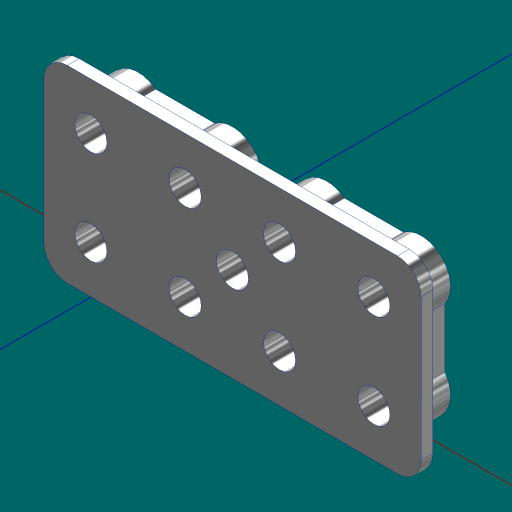
# Autodesk Inventor part: IntakeShoulder
Saved by Autodesk Inventor 2023.1 (Build 271208000, 208)
## iProperties
Created: 2022-11-06
Part Number: IntakeShoulder
Material: Aluminum 6061
Document SubType Name: Modeling
Designer: zac-h
Density: 2.7 g/cm^3
Appearance: Aluminum - Flat
Mass: 11.2632 g
Surface Area: 43.63 cm^2
Volume: 4.17154 cm^3
Author: zac-h
Autodesk Inventor part; units mm, degrees
ref_plane "YZ Plane" through (0, 0, 0) normal (1, 0, 0) x (0, 1, 0)
ref_plane "XZ Plane" through (0, 0, 0) normal (0, 1, 0) x (-1, 0, 0)
ref_plane "XY Plane" through (0, 0, 0) normal (0, 0, 1) x (1, 0, 0)
sketch "Sketch1" plane through (0, 0, 0) normal (0, 0, 1) x (1, 0, 0)
  circle A0 centre (0, 0) radius 2.159
  line L0 (0, 0) -> (38.1, 0) construction
  line L1 (0, 0) -> (0, 12.7) construction
  circle A1 centre (12.7, 0) radius 2.159
  circle A2 centre (25.4, 0) radius 2.159
  circle A3 centre (38.1, 0) radius 2.159
  circle A4 centre (0, 12.7) radius 2.159
  circle A5 centre (12.7, 12.7) radius 2.159
  circle A6 centre (25.4, 12.7) radius 2.159
  circle A7 centre (38.1, 12.7) radius 2.159
  circle A8 centre (19.05, 6.35) radius 2.159
  line L2 (12.7, 12.7) -> (25.4, 0) construction
  line L3 (-6.35, 19.05) -> (44.45, 19.05)
  line L4 (44.45, 19.05) -> (44.45, -6.35)
  line L5 (44.45, -6.35) -> (-6.35, -6.35)
  line L6 (-6.35, -6.35) -> (-6.35, 19.05)
  circle A9 centre (0, 12.7) radius 6.35 construction
  circle A10 centre (38.1, 0) radius 6.35 construction
  dimension "d0" = 4.318
  dimension "d1" = 38.1
  dimension "d9" = 12.7
  dimension "d12" = 12.7
  dimension "d15" = 12.7
  dimension "d18" = 4.318
  dimension "d19" = 25.4
  constraints: 14 end point, 11 centre point, 4 tangent, 3 coincident, 3 horizontal, 2 parallel, 2 vertical, 1 equal radius, 1 midpoint, 1 perpendicular, 14 other
  measures "d0" diameter of A0
  measures "d1" distance of L0.start L0.end
  measures "d9" distance of L0.start L1.end
  measures "d12" distance of L0.start A1.centre
  measures "d15" distance of L0.start A4.centre
  measures "d18" diameter of A8
  measures "d19" distance of L3.end L4.end
extrude "Extrusion1" add sketch "Sketch1" along normal blind 6.35
fillet "Fillet1" radius 3.175 4 edges at (44.45, 19.05, 3.175) (44.45, -6.35, 3.175) (-6.35, -6.35, 3.175) (-6.35, 19.05, 3.175)
sketch "Sketch2" plane through (0, 0, 0) normal (0, 0, -1) x (-1, 0, 0)
  arc A0 (6.35, 15.875) -> (3.175, 19.05) centre (3.175, 15.875) ccw projected
  line L0 (-41.275, 19.05) -> (3.175, 19.05) projected
  arc A1 (-41.275, 19.05) -> (-44.45, 15.875) centre (-41.275, 15.875) ccw projected
  line L1 (-44.45, -3.175) -> (-44.45, 15.875) projected
  arc A2 (-44.45, -3.175) -> (-41.275, -6.35) centre (-41.275, -3.175) ccw projected
  line L2 (3.175, -6.35) -> (-41.275, -6.35) projected
  arc A3 (3.175, -6.35) -> (6.35, -3.175) centre (3.175, -3.175) ccw projected
  line L3 (6.35, 15.875) -> (6.35, -3.175) projected
  circle A4 centre (-19.05, 6.35) radius 2.159 projected
  circle A5 centre (0, 0) radius 2.159 projected
  circle A6 centre (-12.7, 0) radius 2.159 projected
  circle A7 centre (-25.4, 0) radius 2.159 projected
  circle A8 centre (-38.1, 0) radius 2.159 projected
  circle A9 centre (0, 12.7) radius 2.159 projected
  circle A10 centre (-12.7, 12.7) radius 2.159 projected
  circle A11 centre (-25.4, 12.7) radius 2.159 projected
  circle A12 centre (-38.1, 12.7) radius 2.159 projected
  line L4 (3.175, 15.875) -> (3.175, -3.175)
  line L5 (3.175, -3.175) -> (-41.275, -3.175)
  line L6 (-41.275, -3.175) -> (-41.275, 15.875)
  line L7 (-41.275, 15.875) -> (3.175, 15.875)
  circle A13 centre (-38.1, 12.7) radius 3.9688
  circle A14 centre (-25.4, 12.7) radius 3.9688
  circle A15 centre (-12.7, 12.7) radius 3.9688
  circle A16 centre (0, 12.7) radius 3.9688
  circle A17 centre (0, 0) radius 3.9688
  circle A18 centre (-12.7, 0) radius 3.9688
  circle A19 centre (-25.4, 0) radius 3.9688
  circle A20 centre (-38.1, 0) radius 3.9688
  circle A21 centre (-19.05, 6.35) radius 3.9688
  line L8 (-38.1, 12.7) -> (-25.4, 12.7) construction
  line L9 (-38.1, 11.1125) -> (-25.4, 11.1125)
  line L10 (-25.4, 14.2875) -> (-38.1, 14.2875)
  arc A22 (-38.1, 14.2875) -> (-38.1, 11.1125) centre (-38.1, 12.7) ccw
  arc A23 (-25.4, 11.1125) -> (-25.4, 14.2875) centre (-25.4, 12.7) ccw
  line L11 (-25.4, 12.7) -> (-12.7, 0) construction
  line L12 (-26.5225, 11.5775) -> (-13.8225, -1.1225)
  line L13 (-11.5775, 1.1225) -> (-24.2775, 13.8225)
  arc A24 (-24.2775, 13.8225) -> (-26.5225, 11.5775) centre (-25.4, 12.7) ccw
  arc A25 (-13.8225, -1.1225) -> (-11.5775, 1.1225) centre (-12.7, 0) ccw
  line L14 (0, 0) -> (-12.7, 0) construction
  line L15 (0, 1.5875) -> (-12.7, 1.5875)
  line L16 (-12.7, -1.5875) -> (0, -1.5875)
  arc A26 (0, -1.5875) -> (0, 1.5875) centre (0, 0) ccw
  arc A27 (-12.7, 1.5875) -> (-12.7, -1.5875) centre (-12.7, 0) ccw
  line L17 (0, 12.7) -> (-12.7, 12.7) construction
  line L18 (0, 14.2875) -> (-12.7, 14.2875)
  line L19 (-12.7, 11.1125) -> (0, 11.1125)
  arc A28 (0, 11.1125) -> (0, 14.2875) centre (0, 12.7) ccw
  arc A29 (-12.7, 14.2875) -> (-12.7, 11.1125) centre (-12.7, 12.7) ccw
  line L20 (-12.7, 12.7) -> (-25.4, 0) construction
  line L21 (-13.8225, 13.8225) -> (-26.5225, 1.1225)
  line L22 (-24.2775, -1.1225) -> (-11.5775, 11.5775)
  arc A30 (-11.5775, 11.5775) -> (-13.8225, 13.8225) centre (-12.7, 12.7) ccw
  arc A31 (-26.5225, 1.1225) -> (-24.2775, -1.1225) centre (-25.4, 0) ccw
  line L23 (-25.4, 0) -> (-38.1, 0) construction
  line L24 (-25.4, 1.5875) -> (-38.1, 1.5875)
  line L25 (-38.1, -1.5875) -> (-25.4, -1.5875)
  arc A32 (-25.4, -1.5875) -> (-25.4, 1.5875) centre (-25.4, 0) ccw
  arc A33 (-38.1, 1.5875) -> (-38.1, -1.5875) centre (-38.1, 0) ccw
  line L26 (0, 12.7) -> (0, 0) construction
  line L27 (-1.5875, 12.7) -> (-1.5875, 0)
  line L28 (1.5875, 0) -> (1.5875, 12.7)
  arc A34 (1.5875, 12.7) -> (-1.5875, 12.7) centre (0, 12.7) ccw
  arc A35 (-1.5875, 0) -> (1.5875, 0) centre (0, 0) ccw
  line L29 (-38.1, 0) -> (-38.1, 12.7) construction
  line L30 (-36.5125, 0) -> (-36.5125, 12.7)
  line L31 (-39.6875, 12.7) -> (-39.6875, 0)
  arc A36 (-39.6875, 0) -> (-36.5125, 0) centre (-38.1, 0) ccw
  arc A37 (-36.5125, 12.7) -> (-39.6875, 12.7) centre (-38.1, 12.7) ccw
  point P0 (-31.75, 12.7)
  point P1 (-6.35, 0)
  point P2 (-6.35, 12.7)
  point P3 (-19.05, 6.35)
  point P4 (-31.75, 0)
  point P5 (0, 6.35)
  point P6 (-38.1, 6.35)
  point P7 (-20.4995, 2.6554)
  point P8 (-21.7054, 1.4495)
  point P9 (-23.0187, -3.175)
  point P10 (-15.0812, -3.175)
  point P11 (-16.3946, 1.4495)
  point P12 (-17.6005, 2.6554)
  point P13 (-1.5875, 3.6374)
  point P14 (-1.5875, 9.0626)
  point P15 (-3.6374, 11.1125)
  point P16 (-9.0626, 11.1125)
  point P17 (-14.1495, 9.0054)
  point P18 (-15.3554, 7.7995)
  point P19 (-15.3554, 4.9005)
  point P20 (-14.1495, 3.6946)
  point P21 (-9.0626, 1.5875)
  point P22 (-3.6374, 1.5875)
  point P23 (-17.6005, 10.0446)
  point P24 (-16.3946, 11.2505)
  point P25 (-15.0812, 15.875)
  point P26 (-23.0187, 15.875)
  point P27 (-21.7054, 11.2505)
  point P28 (-20.4995, 10.0446)
  point P29 (-36.5125, 9.0626)
  point P30 (-36.5125, 3.6374)
  point P31 (-34.4626, 1.5875)
  point P32 (-29.0374, 1.5875)
  point P33 (-23.9505, 3.6946)
  point P34 (-22.7446, 4.9005)
  point P35 (-22.7446, 7.7995)
  point P36 (-23.9505, 9.0054)
  point P37 (-29.0374, 11.1125)
  point P38 (-34.4626, 11.1125)
  point P39 (-41.275, 2.3812)
  point P40 (-41.275, 10.3188)
  point P41 (-35.7187, 15.875)
  point P42 (-27.7812, 15.875)
  point P43 (-10.3187, 15.875)
  point P44 (-2.3813, 15.875)
  point P45 (3.175, 10.3188)
  point P46 (3.175, 2.3812)
  point P47 (-2.3813, -3.175)
  point P48 (-10.3187, -3.175)
  point P49 (-27.7812, -3.175)
  point P50 (-35.7188, -3.175)
  dimension "d23" = 3.175
  dimension "d25" = 7.9375
  dimension "d27" = 3.175
  dimension "d28" = 3.175
  dimension "d29" = 3.175
  dimension "d30" = 3.175
  dimension "d31" = 3.175
  dimension "d32" = 3.175
  dimension "d33" = 3.175
  dimension "d35" = 3.175
  constraints: 72 end point, 32 point on circle, 32 tangent, 25 centre point, 11 parallel, 9 equal radius, 8 coincident, 8 midpoint, 2 perpendicular, 2 point on line, 1 horizontal, 3 other
  measures "d23" distance between parallel lines of L0 L7
  measures "d25" diameter of A13
  measures "d27" diameter of A23
  measures "d28" diameter of A25
  measures "d29" diameter of A27
  measures "d30" diameter of A29
  measures "d31" diameter of A31
  measures "d32" diameter of A33
  measures "d33" diameter of A35
  measures "d35" distance between parallel lines of L31 L30
extrude "Extrusion2" cut sketch "Sketch2" against normal blind 4.7625 contours L3 A3 L2 A2 L1 A1 L0 A0 | A21 L22 A15 L19 A16 L27 A17 L15 A18 L13 | L13 A14 L7 A15 L21 A21 | L12 A18 L5 A19 L22 A21 | A21 L21 A19 L24 A20 L30 A13 L9 A14 L12 | L7 L4 A16 | A17 L4 L5 | A13 L6 L7 | L5 L6 A20
fillet "Fillet2" radius 1.75 28 edges at (34.4626, 11.1125, 2.3813) (36.5125, 9.0626, 2.3813) (36.5125, 3.6374, 2.3813) (34.4626, 1.5875, 2.3813) (29.0374, 1.5875, 2.3813) (23.9505, 3.6946, 2.3813) (22.7446, 4.9005, 2.3813) (22.7446, 7.7995, 2.3813) (23.9505, 9.0054, 2.3813) (29.0374, 11.1125, 2.3813) (21.7054, 11.2505, 2.3813) (20.4995, 10.0446, 2.3813) (17.6005, 10.0446, 2.3813) (16.3946, 11.2505, 2.3813) (9.0626, 11.1125, 2.3813) (3.6374, 11.1125, 2.3813) (1.5875, 9.0626, 2.3813) (1.5875, 3.6374, 2.3813) (3.6374, 1.5875, 2.3813) (9.0626, 1.5875, 2.3813) (14.1495, 3.6946, 2.3813) (15.3554, 4.9005, 2.3813) (15.3554, 7.7995, 2.3813) (14.1495, 9.0054, 2.3813) (20.4995, 2.6554, 2.3813) (17.6005, 2.6554, 2.3813) (16.3946, 1.4495, 2.3813) (21.7054, 1.4495, 2.3813)
body "Solid1"
